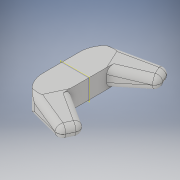
# Autodesk Inventor part: contour phase
Saved by Autodesk Inventor 2018 (Build 220112000, 112)
## iProperties
Created: 2017-08-07
Part Number: contour phase
Material: Generic
Document SubType Name: Modeling
Designer: asmith50
Density: 1 g/cm^3
Appearance: Default
Author: asmith50
Autodesk Inventor part; units mm, degrees
ref_plane "YZ Plane" through (0, 0, 0) normal (1, 0, 0) x (0, 1, 0)
ref_plane "XZ Plane" through (0, 0, 0) normal (0, 1, 0) x (-1, 0, 0)
ref_plane "XY Plane" through (0, 0, 0) normal (0, 0, 1) x (1, 0, 0)
sketch "Sketch1" plane through (0, 0, 0) normal (0, 1, 0) x (-1, 0, 0)
  line L0 (0, 0) -> (-70, 0)
  line L1 (-70, 0) -> (-70, -95)
  line L2 (-70, -95) -> (0, -95)
  line L3 (0, -95) -> (0, 0)
  dimension "d0" = 70
  dimension "d1" = 95
  constraints: 8 end point, 2 parallel, 1 horizontal, 1 perpendicular
  measures "d0" distance of L2.end L1.end
  measures "d1" distance of L1.end L0.end
extrude "Extrusion1" add sketch "Sketch1" along normal blind 50
sketch "Sketch2" plane through (0, 0, 0) normal (0, 0, 1) x (1, 0, 0)
  line L0 (0, 50) -> (70, 50) projected
  line L1 (0, 0) -> (70, 0)
  line L2 (70, 0) -> (70, 50)
  line L3 (70, 50) -> (0, 50)
  line L4 (0, 50) -> (0, 0)
  constraints: 8 end point, 2 parallel, 1 horizontal, 1 perpendicular
revolve "Revolution1" add sketch "Sketch2" angle 65 about axis through (70, 0, 0) along (0, 1, 0)
sketch "Sketch3" plane through (70, 0, 0) normal (0.9063078, 0, 0.4226183) x (0.4226183, 0, -0.9063078)
  line L0 (-29.5833, 50) -> (-70, 50) projected
  line L1 (-70, 0) -> (0, 0) projected
  line L2 (-70, 50) -> (0, 50)
  line L3 (0, 50) -> (0, 0)
  line L4 (0, 0) -> (-70, 0)
  line L5 (-70, 0) -> (-70, 50)
  point P0 (-29.5833, 0)
  constraints: 8 end point, 2 parallel, 1 horizontal, 1 perpendicular
extrude "Extrusion2" add sketch "Sketch3" along normal blind 100 draft -6
ref_plane "Work Plane1" through (70, 0, -47.5) normal (0, 0, -1) x (-1, 0, 0)
mirror "Mirror1" about plane through (70, 0, -47.5) normal (0, 0, -1) of "Revolution1", "Extrusion2"
fillet "Fillet1" radius 16.002 16 edges at (87.9531, 44.7448, 79.8096) (113.0944, 44.7448, 25.8938) (145.8391, 39.4896, 73.9826) (145.8391, 10.5104, 73.9826) (135.4894, 25, 96.1777) (156.1889, 25, 51.7875) (87.9531, 5.2552, 79.8096) (113.0944, 5.2552, 25.8938) (113.0944, 5.2552, -120.8938) (113.0944, 44.7448, -120.8938) (156.1889, 25, -146.7875) (145.8391, 39.4896, -168.9826) (145.8391, 10.5104, -168.9826) (87.9531, 5.2552, -174.8096) (135.4894, 25, -191.1777) (87.9531, 44.7448, -174.8096)
body "Solid1"
